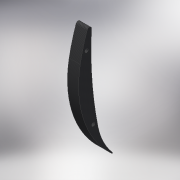
# Autodesk Inventor part: styro_50_main
Saved by Autodesk Inventor 2018.2 (Build 222227000, 227)
## iProperties
Created: 2017-12-11
Part Number: styro_50_main
Material: ポリスチレン、耐衝撃性
Document SubType Name: Modeling
Designer: kuwano
Density: 1.022 g/cm^3
Appearance: カーボンファイバー
Mass: 1214.74 g
Surface Area: 1128.2 cm^2
Volume: 1188.59 cm^3
Author: kuwano
Autodesk Inventor part; units mm, degrees
ref_plane "YZ Plane" through (0, 0, 0) normal (1, 0, 0) x (0, 1, 0)
ref_plane "XZ Plane" through (0, 0, 0) normal (0, 1, 0) x (-1, 0, 0)
ref_plane "XY Plane" through (0, 0, 0) normal (0, 0, 1) x (1, 0, 0)
sketch "スケッチ1" plane through (0, 0, 0) normal (1, 0, 0) x (0, 1, 0)
  line L0 (-3.1158, 220) -> (114.6125, -400)
  line L1 (-4.9236, 357.8045) -> (7.4936, -588.754)
  arc A0 (-3.1158, 220) -> (21.0831, -240) centre (1567.8058, 72.0039) ccw
  arc A1 (21.0831, -240) -> (114.6125, -400) centre (301.453, -183.444) ccw
  arc A2 (-3.1158, 220) -> (-58.3522, 40.8591) centre (728.4844, -103.6681) ccw
  arc A3 (-58.3522, 40.8591) -> (114.6125, -400) centre (383.2315, -40.2516) ccw
  point P0 (0, 0)
  point P1 (-3.1158, -30)
  point P2 (-4.9236, 357.8045)
  dimension "d0" = 10
  dimension "d1" = 620
  dimension "d2" = 250
  dimension "d3" = 1577.8776
  dimension "d4" = 286.0172
  dimension "d5" = 160
  dimension "d6" = 800
  constraints: 8 point on circle, 4 centre point, 2 end point, 2 tangent, 4 other
  measures "d1" vertical distance of L0.end L0.start
  measures "d2" distance of point (-3.116, -30) L0.start
  measures "d3" radius of A0
  measures "d4" radius of A1
  measures "d5" vertical distance of L0.end A0.end
  measures "d6" radius of A2
extrude "押し出し1" add sketch "スケッチ1" along normal mid plane 50 contours A0 L1 A3 A2 | A3 L1 A0 A1
fillet "フィレット1" radius 10 1 edges at (0, -3.1158, 220)
fillet "フィレット1" radius 2 1 edges at (0, 114.6125, -400)
sketch "スケッチ2" plane through (25, 0, 0) normal (1, 0, 0) x (0, 0, -1)
  circle A0 centre (-80, -30) radius 7.5
  circle A1 centre (220, 0) radius 7.5
  point P0 (0, 0)
  dimension "d11" = 15
  dimension "d12" = 15
  dimension "d13" = 300
  dimension "d16" = 30
  dimension "d19" = 30
  dimension "d20" = 80
  constraints: 2 centre point
  measures "d11" diameter of A1
  measures "d12" diameter of A0
  measures "d13" horizontal distance of A1.centre A0.centre
  measures "d16" vertical distance of A1.centre A0.centre
  measures "d19" vertical distance of A0.centre point (0, 0)
  measures "d20" horizontal distance of A0.centre point (0, 0)
extrude "押し出し2" cut sketch "スケッチ2" against normal through all
